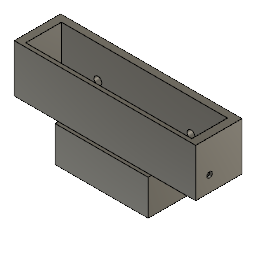
switch enclosure V4 (Autodesk Fusion 360 design; units mm, degrees)
Autodesk Fusion 360 part; units mm, degrees
sketch "Main Profile" plane through (0, 0, 0) normal (0, 0, 1) x (1, 0, 0)
  line L0 (30, 17) -> (-30, 17)
  line L1 (-30, 17) -> (-30, -17)
  line L2 (-30, -17) -> (30, -17)
  line L3 (30, -17) -> (30, 17)
  line L4 (30, 17) -> (-30, -17) construction
  line L5 (-30, 17) -> (30, -17) construction
  line L6 (-22.875, 10) -> (22.875, 10)
  line L7 (22.875, 10) -> (22.875, -10)
  line L8 (22.875, -10) -> (-22.875, -10)
  line L9 (-22.875, -10) -> (-22.875, 10)
  line L10 (-22.875, 10) -> (22.875, -10) construction
  line L11 (22.875, 10) -> (-22.875, -10) construction
  line L12 (24.75, -12) -> (-24.75, -12)
  line L13 (-24.75, -12) -> (-24.75, 12)
  line L14 (-24.75, 12) -> (24.75, 12)
  line L15 (24.75, 12) -> (24.75, -12)
  line L16 (24.75, -12) -> (-24.75, 12) construction
  line L17 (-24.75, -12) -> (24.75, 12) construction
  line L18 (-58.5, 15.1) -> (58.5, 15.1)
  line L19 (58.5, 15.1) -> (58.5, -14.9)
  line L20 (58.5, -14.9) -> (-58.5, -14.9)
  line L21 (-58.5, -14.9) -> (-58.5, 15.1)
  line L22 (-53.5, 10.6) -> (53.5, 10.6)
  line L23 (53.5, 10.6) -> (53.5, -12.4)
  line L24 (53.5, -12.4) -> (-53.5, -12.4)
  line L25 (-53.5, -12.4) -> (-53.5, 10.6)
  line L26 (28, -14.9) -> (-28, -14.9)
  line L27 (-28, -14.9) -> (-28, 14.9)
  line L28 (-28, 14.9) -> (28, 14.9)
  line L29 (28, 14.9) -> (28, -14.9)
  line L30 (28, -14.9) -> (-28, 14.9) construction
  line L31 (-28, -14.9) -> (28, 14.9) construction
  dimension "d1" = 60
  dimension "d2" = 34
  dimension "d3" = 45.75
  dimension "d4" = 20
  dimension "d5" = 49.5
  dimension "d6" = 24
  dimension "d7" = 117
  dimension "d8" = 30
  dimension "d9" = 23
  dimension "d10" = 107
  dimension "d11" = 12.4
  dimension "d12" = 53.5
  dimension "d13" = 2.5
  dimension "d14" = 5
  dimension "d15" = 56
  constraint perpendicular L0 L1
  constraint parallel L0 L2
  constraint parallel L1 L3
  constraint horizontal L0
  constraint coincident L4 origin
  constraint coincident L5 origin
  constraint perpendicular L6 L7
  constraint parallel L6 L8
  constraint parallel L7 L9
  constraint horizontal L6
  constraint coincident L10 origin
  constraint coincident L11 origin
  constraint perpendicular L12 L13
  constraint parallel L12 L14
  constraint parallel L13 L15
  constraint horizontal L12
  constraint coincident L16 origin
  constraint coincident L17 origin
  constraint horizontal L18
  constraint vertical L19
  constraint horizontal L20
  constraint vertical L21
  constraint horizontal L22
  constraint vertical L23
  constraint horizontal L24
  constraint vertical L25
  constraint perpendicular L26 L27
  constraint parallel L26 L28
  constraint parallel L27 L29
  constraint horizontal L26
  constraint coincident L20 L26.start
  constraint coincident L30 origin
  constraint coincident L31 origin
  measures "d1" distance of L1.end L2.end
  measures "d2" distance of L0.end L1.end
  measures "d3" distance of L7.end L8.end
  measures "d4" distance of L6.end L7.end
  measures "d5" distance of L13.end L14.end
  measures "d6" distance of L12.end L13.end
  measures "d7" distance of L18.start L18.end
  measures "d8" distance of L18.start L20.end
  measures "d9" distance of L22.start L24.end
  measures "d10" distance of L22.start L22.end
  measures "d11" distance of origin L24
  measures "d12" distance of origin L25
  measures "d13" distance of L20 L24
  measures "d14" distance of L21 L25
  measures "d15" distance of L26.start L26.end
extrude "Extrude1" add sketch "Main Profile" along normal blind 23 contours L0 L1 L3 L18 | L1 L3 L18 L22 L27 L28 L29 | L3 L22 L24 L29 | L1 L22 L24 L27 | L3 L20 L24 L29 | L1 L20 L24 L27 | L1 L2 L3 L20 L26
extrude "Extrude2" add sketch "Main Profile" along normal blind 5 contours L12 L13 L15 L22 L24 L27 L29 | L13 L14 L15 L22 L27 L28 L29 | L20 L24 L26 L27 L29
extrude "Extrude3" add sketch "Main Profile" along normal blind 1.5 from surface at 3.5 contours L13 L14 L15 L22 | L12 L13 L15 L22
extrude "Extrude4" add sketch "Main Profile" along normal blind 2 from surface at 23 contours L3 L18 L19 L20 L22 L23 L24 | L1 L3 L18 L22 L27 L28 L29 | L1 L18 L20 L21 L22 L24 L25 | L3 L22 L23 L24 | L3 L22 L24 L29 | L1 L22 L24 L27 | L1 L22 L24 L25 | L3 L20 L24 L29 | L13 L14 L15 L22 L27 L28 L29 | L1 L20 L24 L27 | L20 L24 L26 L27 L29 | L13 L14 L15 L22
extrude "Extrude5" add sketch "Main Profile" along normal blind 29 from surface at 25 contours L3 L18 L19 L20 L22 L23 L24 | L1 L3 L18 L22 L27 L28 L29 | L1 L18 L20 L21 L22 L24 L25 | L3 L20 L24 L29 | L13 L14 L15 L22 L27 L28 L29 | L1 L20 L24 L27 | L20 L24 L26 L27 L29 | L13 L14 L15 L22
sketch "EndHoles" plane through (58.5, 0, 0) normal (1, 0, 0) x (0, 1, 0)
  line L0 (-14.9, 23) -> (15.1, 23)
  line L1 (15.1, 23) -> (15.1, 54)
  line L2 (15.1, 54) -> (-14.9, 54)
  line L3 (-14.9, 54) -> (-14.9, 23)
  circle A0 centre (-5.9, 33.1) radius 2.5
  circle A1 centre (-5.9, 33.1) radius 1.75
  dimension "d29" = 5
  dimension "d30" = 3.5
  dimension "d31" = 9
  dimension "d32" = 20.9
  constraint concentric A0 A1
  measures "d29" diameter of A0
  measures "d30" diameter of A1
  measures "d31" distance of L3 A0.centre
  measures "d32" distance of L2 A0.centre
extrude "Extrude6" cut sketch "EndHoles" against normal blind 136.67 contours A1
extrude "Extrude7" cut sketch "EndHoles" along normal blind 3.5 from surface at -5 contours A0
extrude "Extrude8" cut sketch "EndHoles" against normal blind 3.5 from surface at -112 contours A0
sketch "SideHoles" plane through (0, 10.6, 0) normal (0, -1, 0) x (1, 0, 0)
  line L0 (-28, 23) -> (28, 23)
  line L1 (28, 23) -> (28, 25)
  line L2 (28, 25) -> (53.5, 25)
  line L3 (53.5, 25) -> (53.5, 54)
  line L4 (53.5, 54) -> (-53.5, 54)
  line L5 (-53.5, 54) -> (-53.5, 25)
  line L6 (-53.5, 25) -> (-28, 25)
  line L7 (-28, 25) -> (-28, 23)
  circle A0 centre (-30, 33.1) radius 2.5
  circle A1 centre (-30, 33.1) radius 1.75
  circle A2 centre (30, 33.1) radius 1.75
  circle A3 centre (30, 33.1) radius 2.5
  dimension "d41" = 5
  dimension "d42" = 3.5
  dimension "d43" = 20.9
  dimension "d44" = 23.5
  dimension "d47" = 60
  dimension "d48" = 0
  constraint concentric A0 A1
  measures "d41" diameter of A0
  measures "d42" diameter of A1
  measures "d43" distance of L4 A0.centre
  measures "d44" distance of L5 A0.centre
extrude "Extrude9" cut sketch "SideHoles" against normal blind 10 contours A1 | A2
extrude "Extrude10" cut sketch "SideHoles" against normal blind 3.5 contours A0 | A3
chamfer "Chamfer1" distance 1.5 distance2 3 1 edges at (0, 14.9, 23) measured on face at (-9.3333, 13.4667, 23)
mirror "Mirror1" about plane through (0, 0, 0) normal (0, 1, 0) of 1 faces at (-9.3333, 14.4, 21)
named bodies: "switch enclosure V4"
